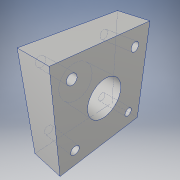
# Autodesk Inventor part: Joint Mount
Saved by Autodesk Inventor 2019 (Build 230136000, 136)
## iProperties
Created: 2018-09-25
Part Number: Joint Mount
Material: Aluminum 6061
Document SubType Name: Modeling
Designer: Adhik
Density: 2.7 g/cm^3
Appearance: Aluminum - Flat
Author: Adhik
Autodesk Inventor part; units mm, degrees
ref_plane "YZ Plane" through (0, 0, 0) normal (1, 0, 0) x (0, 1, 0)
ref_plane "XZ Plane" through (0, 0, 0) normal (0, 1, 0) x (-1, 0, 0)
ref_plane "XY Plane" through (0, 0, 0) normal (0, 0, 1) x (1, 0, 0)
sketch "Sketch1" plane through (0, 0, 0) normal (1, 0, 0) x (0, 1, 0)
  line L0 (0, -26.67) -> (0, 26.67) construction
  line L1 (-26.67, 0) -> (26.67, 0) construction
  line L2 (19.05, 19.05) -> (-19.05, 19.05)
  line L3 (-19.05, 19.05) -> (-19.05, -19.05)
  line L4 (-19.05, -19.05) -> (19.05, -19.05)
  line L5 (19.05, -19.05) -> (19.05, 19.05)
  circle A0 centre (0, 0) radius 7.3422
  line L6 (12.7, 12.7) -> (-12.7, 12.7) construction
  line L7 (-12.7, 12.7) -> (-12.7, -12.7) construction
  line L8 (-12.7, -12.7) -> (12.7, -12.7) construction
  line L9 (12.7, -12.7) -> (12.7, 12.7) construction
  circle A1 centre (12.7, 12.7) radius 1.778
  circle A2 centre (12.7, -12.7) radius 1.778
  circle A3 centre (-12.7, -12.7) radius 1.778
  circle A4 centre (-12.7, 12.7) radius 1.778
  point P0 (19.05, 0)
  point P1 (0, 19.05)
  point P2 (12.7, 0)
  point P3 (0, 12.7)
  dimension "d0" = 38.1
  dimension "d1" = 14.6844
  dimension "d2" = 3.556
  dimension "d3" = 25.4
  constraints: 16 end point, 5 centre point, 5 coincident, 4 midpoint, 4 parallel, 4 perpendicular, 4 point on line, 3 equal radius, 2 horizontal
  measures "d0" distance of L2.start L2.end
  measures "d1" diameter of A0
  measures "d2" diameter of A1
  measures "d3" distance of L8.end L6.start
extrude "Extrusion1" add sketch "Sketch1" along normal blind 12.7
body "Solid1"
